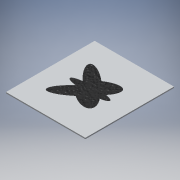
# Autodesk Inventor part: Butterfly Logo plexiglass plane
Saved by Autodesk Inventor 2019 (Build 230136000, 136)
## iProperties
Created: 2019-02-07
Part Number: Butterfly Logo plexiglass plane
Material: Generic
Document SubType Name: Modeling
Designer: mrhftc
Density: 1 g/cm^3
Appearance: Default
Author: mrhftc
Autodesk Inventor part; units mm, degrees
ref_plane "YZ Plane" through (0, 0, 0) normal (1, 0, 0) x (0, 1, 0)
ref_plane "XZ Plane" through (0, 0, 0) normal (0, 1, 0) x (-1, 0, 0)
ref_plane "XY Plane" through (0, 0, 0) normal (0, 0, 1) x (1, 0, 0)
sketch "Sketch1" plane through (0, 0, 0) normal (0, 1, 0) x (-1, 0, 0)
  line L0 (94.6629, 106.9998) -> (-121.2371, 106.9998)
  line L1 (-121.2371, 106.9998) -> (-121.2371, -134.3002)
  line L2 (-121.2371, -134.3002) -> (94.6629, -134.3002)
  line L3 (94.6629, -134.3002) -> (94.6629, 106.9998)
  point P0 (0, 0)
  dimension "d0" = 241.3
  dimension "d1" = 215.9
  constraints: 8 end point, 2 parallel, 1 horizontal, 1 perpendicular
  measures "d0" distance between parallel lines of L2 L0
  measures "d1" distance between parallel lines of L1 L3
extrude "Extrusion1" add sketch "Sketch1" along normal blind 3.175
sketch "Sketch2" plane through (0, 3.175, 0) normal (0, 1, 0) x (1, 0, 0)
  ellipse E0 centre (0, 32.9329) end of major axis (-46.7996, 73.8447) minor radius 18.0599 (9.3407, 48.7201) -> (-16.3986, 23.3952) ccw
  ellipse E1 centre (17.4405, 25.2301) end of major axis (58.9723, 57.8521) minor radius 23.76 (48.6403, 22.4972) -> (9.3407, 48.7201) ccw
  ellipse E2 centre (17.4405, 25.2301) end of major axis (58.9723, 57.8521) minor radius 23.76 (-16.9368, 23.8952) -> (-17.4025, 23.2533) ccw
  ellipse E3 centre (13.2871, 13.6502) end of major axis (-41.2842, 13.6502) minor radius 11.6136 (-16.3986, 23.3952) -> (-41.2842, 13.6502) ccw
  ellipse E4 centre (13.2871, 13.6502) end of major axis (-41.2842, 13.6502) minor radius 11.6136 (67.8584, 13.6502) -> (48.6403, 22.4972) ccw
  ellipse E5 centre (0, -5.6325) end of major axis (-46.7996, -46.5443) minor radius 18.0599 (-16.3986, 3.9052) -> (9.3407, -21.4198) ccw
  ellipse E6 centre (17.4405, 2.0702) end of major axis (58.9723, -30.5517) minor radius 23.76 (9.3407, -21.4198) -> (48.6403, 4.8031) ccw
  ellipse E7 centre (17.4405, 2.0702) end of major axis (58.9723, -30.5517) minor radius 23.76 (-17.4025, 4.0471) -> (-16.9368, 3.4052) ccw
  ellipse E8 centre (13.2871, 13.6502) end of major axis (-41.2842, 13.6502) minor radius 11.6136 (-41.2842, 13.6502) -> (-16.3986, 3.9052) ccw
  ellipse E9 centre (13.2871, 13.6502) end of major axis (-41.2842, 13.6502) minor radius 11.6136 (48.6403, 4.8031) -> (67.8584, 13.6502) ccw
  point P0 (0, 0)
  constraints: 42 other
extrude "Extrusion2" cut sketch "Sketch2" against normal blind 0.635 contours E1 E4 E9 E6 E5 E8 E3 E0
body "Solid1"
